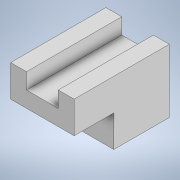
# Autodesk Inventor part: 5
Saved by Autodesk Inventor 2022 (Build 260153000, 153)
## iProperties
Created: 2022-03-14
Part Number: 5
Material: Všeobecné
Document SubType Name: Modeling
Designer: Šimon
Density: 1 g/cm^3
Appearance: Výchozí
Author: Šimon
Autodesk Inventor part; units mm, degrees
ref_plane "YZ Plane" through (0, 0, 0) normal (1, 0, 0) x (0, 1, 0)
ref_plane "XZ Plane" through (0, 0, 0) normal (0, 1, 0) x (-1, 0, 0)
ref_plane "XY Plane" through (0, 0, 0) normal (0, 0, 1) x (1, 0, 0)
sketch "Náčrt1" plane through (0, 0, 0) normal (0, 0, 1) x (1, 0, 0)
  line L0 (0, 0) -> (40, 0)
  line L1 (40, 0) -> (40, 40)
  line L2 (40, 40) -> (30, 40)
  line L3 (30, 40) -> (30, 30)
  line L4 (30, 30) -> (10, 30)
  line L5 (10, 30) -> (10, 40)
  line L6 (10, 40) -> (0, 40)
  line L7 (0, 40) -> (0, 0)
  dimension "d0" = 40
  dimension "d1" = 40
  dimension "d2" = 10
  dimension "d3" = 10
  dimension "d4" = 20
  dimension "d5" = 10
  dimension "d6" = 10
  constraints: 16 end point, 5 perpendicular, 1 horizontal, 1 vertical
  measures "d0" distance of L0.start L0.end
  measures "d1" distance of L0.end L1.end
  measures "d2" distance of L1.end L2.end
  measures "d3" distance of L2.end L3.end
  measures "d4" distance of L3.end L4.end
  measures "d5" distance of L4.end L5.end
  measures "d6" distance of L5.end L6.end
extrude "Vysunutí1" add sketch "Náčrt1" against normal blind 60
sketch "Náčrt2" plane through (0, 0, 0) normal (0, 0, 1) x (1, 0, 0)
  line L0 (40, 0) -> (0, 0) projected
  line L1 (40, 0) -> (40, 20)
  line L2 (40, 0) -> (40, 40) projected
  line L3 (40, 20) -> (20, 20)
  line L4 (20, 20) -> (20, 0)
  line L5 (20, 0) -> (40, 0)
  dimension "d11" = 20
  dimension "d12" = 20
  constraints: 8 end point, 3 perpendicular, 1 midpoint
  measures "d11" distance of L0.start L1.end
  measures "d12" distance of L1.end L3.end
extrude "Vysunutí2" cut sketch "Náčrt2" against normal blind 25
sketch "Náčrt3" plane through (0, 0, 0) normal (-1, 0, 0) x (0, 0, 1)
  line L0 (0, 40) -> (0, 0) projected
  line L1 (-25, 0) -> (0, 0) projected
  line L2 (0, 0) -> (-25, 0)
  line L3 (0, 20) -> (-25, 0)
  line L4 (0, 0) -> (0, 20)
  constraints: 6 end point, 2 collinear
extrude "Vysunutí3" cut sketch "Náčrt3" against normal blind 25
